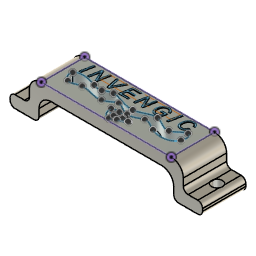
Handle (Autodesk Fusion 360 design; units mm, degrees)
part number: 2025-07-22-14-27-28-106
Autodesk Fusion 360 part; units mm, degrees
note: some values were not read from the file. Chosen so that the rebuilt part matches the saved one: which bodies a step acts on. Set by a fixed rule: which sketch regions a step uses.
sketch "Sketch1" plane through (0, 0, 0) normal (0, 1, 0) x (1, 0, 0)
  line L0 (-40, -2) -> (-40, -3)
  line L1 (-38, -5) -> (-34, -5)
  line L2 (-32, -7) -> (-32, -10)
  line L3 (-27, -15) -> (0.0378, -15)
  line L4 (0, -1.75) -> (0, -22.5)
  line L5 (0, 0) -> (38, 0)
  line L6 (40, -2) -> (40, -3)
  line L7 (38, -5) -> (34, -5)
  line L8 (32, -7) -> (32, -10)
  line L9 (27, -15) -> (-0.0378, -15)
  line L10 (-38, 0) -> (-30, 0)
  line L11 (-28, -2) -> (-28, -5)
  line L12 (-23, -10) -> (0, -10)
  line L13 (40, 0) -> (30, 0)
  line L14 (28, -2) -> (28, -5)
  line L15 (23, -10) -> (0, -10)
  arc A0 (-32, -10) -> (-27, -15) centre (-27, -10) ccw
  arc A1 (27, -15) -> (32, -10) centre (27, -10) ccw
  arc A2 (-28, -5) -> (-23, -10) centre (-23, -5) ccw
  arc A3 (23, -10) -> (28, -5) centre (23, -5) ccw
  arc A4 (-38, 0) -> (-40, -2) centre (-38, -2) ccw
  arc A5 (40, -2) -> (38, 0) centre (38, -2) ccw
  arc A6 (38, -5) -> (40, -3) centre (38, -3) ccw
  arc A7 (30, 0) -> (28, -2) centre (30, -2) ccw
  arc A8 (-28, -2) -> (-30, 0) centre (-30, -2) ccw
  arc A9 (-32, -7) -> (-34, -5) centre (-34, -7) ccw
  arc A10 (34, -5) -> (32, -7) centre (34, -7) ccw
  arc A11 (-40, -3) -> (-38, -5) centre (-38, -3) ccw
  point P0 (-40, 0)
  point P1 (-40, -5)
  point P2 (-32, -5)
  point P3 (-32, -15)
  point P4 (-28, 0)
  dimension "d7" = 40
  dimension "d8" = 5
  dimension "d9" = 8
  dimension "d10" = 10
  dimension "d18" = 12
  dimension "d41" = 5
  dimension "d53" = 5
  dimension "d54" = 5
  dimension "d55" = 2
  dimension "d56" = 2
  constraint perpendicular L0 L1
  constraint perpendicular L1 L2
  constraint perpendicular L2 L3
  constraint symmetric L3.end L4 L9.end
  constraint perpendicular L0 L10
  constraint perpendicular L10 L11
  constraint coincident L4 L12.end
  constraint perpendicular L4 L12
  constraint symmetric P0 L4 L13.start
  constraint symmetric L4 L12.end L15.end
  constraint coincident P3 L2
  constraint coincident P3 L3
  constraint tangent L2 A0
  constraint tangent L3 A0
  constraint symmetric L4 L2.end L8.end
  constraint symmetric L4 L3.start L9.start
  constraint symmetric L4 A0 A1
  constraint tangent L11 A2
  constraint tangent L12 A2
  constraint tangent L14 A3
  constraint tangent L15 A3
  constraint equal A2 A3
  constraint coincident P0 L0
  constraint coincident P0 L10
  constraint tangent L0 A4
  constraint tangent L10 A4
  constraint tangent L5 A5
  constraint tangent L6 A5
  constraint equal A4 A5
  constraint tangent L6 A6
  constraint tangent L7 A6
  constraint equal A4 A6
  constraint tangent L13 A7
  constraint tangent L14 A7
  constraint equal A4 A7
  constraint coincident P4 L10
  constraint coincident P4 L11
  constraint tangent L10 A8
  constraint tangent L11 A8
  constraint equal A4 A8
  constraint coincident P2 L1
  constraint coincident P2 L2
  constraint tangent L1 A9
  constraint tangent L2 A9
  constraint equal A4 A9
  constraint tangent L7 A10
  constraint tangent L8 A10
  constraint equal A4 A10
  constraint coincident P1 L0
  constraint coincident P1 L1
  constraint tangent L0 A11
  constraint tangent L1 A11
  measures "d7" distance of L5.start P0
  measures "d8" distance of P0 P1
  measures "d9" distance of P1 P2
  measures "d10" distance of P2 P3
  measures "d18" distance of P0 P4
  measures "d41" distance of L3 L12
  measures "d53" radius of A0
  measures "d54" radius of A2
  measures "d55" radius of A4
  measures "d56" radius of A11
extrude "Extrude2" add sketch "Sketch1" along normal blind 18 makes body 1
sketch "Sketch3" plane through (0, 0, 15) normal (0, 0, 1) x (-1, 0, 0)
  line L0 (27, 0) -> (-27, 0)
  line L1 (-27, -18) -> (27, -18)
  line L2 (15.4669, -13.2004) -> (-13.5401, -13.4911) construction
  line L3 (-13.5401, -13.4911) -> (-13.5035, -17.1453) construction
  line L4 (-13.5035, -17.1453) -> (15.5035, -16.8547) construction
  line L5 (15.5035, -16.8547) -> (15.4669, -13.2004) construction
  spline S0 degree 5 poles (3, -5) (3, -4.7009) (2.9694, -4.1277) (2.8315, -3.3428) (2.4733, -2.45) (1.7882, -1.6139) (0.9367, -1.0903) (0, -0.9102) (-0.9367, -1.0903) (-1.7882, -1.6139) (-2.4733, -2.45) (-2.8315, -3.3428) (-2.9694, -4.1277) (-3, -4.7009) (-3, -5) knots 0 0 0 0 0 0 0.1 0.2 0.3 0.4 0.5 0.6 0.7 0.8 0.9 1 1 1 1 1 1
  line L6 (3, -6) -> (3, -4)
  line L7 (-3, -4) -> (-3, -6)
  spline S1 degree 5 poles (3, -5) (3.0104, -4.9295) (3.0012, -4.7732) (2.8966, -4.496) (2.5814, -4.0664) (1.9381, -3.5344) (1.1107, -3.1246) (0.179, -2.9363) (-0.7694, -3.0239) (-1.6457, -3.3607) (-2.3664, -3.8604) (-2.8601, -4.409) (-3.0745, -4.894) (-2.983, -5.2313) (-2.5948, -5.4017) (-1.9522, -5.4436) (-1.1205, -5.4206) (-0.1814, -5.3963) (0.7751, -5.4088) (1.6575, -5.4391) (2.3801, -5.4296) (2.7723, -5.3367) (2.9386, -5.1964) (2.9896, -5.0705) (3, -5) knots 0 0 0 0 0 0 0.05 0.1 0.15 0.2 0.25 0.3 0.35 0.4 0.45 0.5 0.55 0.6 0.65 0.7 0.75 0.8 0.85 0.9 0.95 1 1 1 1 1 1
  spline S2 degree 5 poles (-1.9403, -1.8799) (-2.1918, -1.9781) (-2.6753, -2.1699) (-3.3422, -2.4439) (-4.1125, -2.7815) (-4.8632, -3.1539) (-5.3805, -3.4718) (-5.6414, -3.7297) (-5.6271, -3.9233) (-5.3382, -4.0528) (-4.7908, -4.1218) (-4.161, -4.1322) (-3.5872, -4.1163) (-3.1604, -4.0953) (-2.9358, -4.0822) knots 0 0 0 0 0 0 0.1 0.2 0.3 0.4 0.5 0.6 0.7 0.8 0.9 1 1 1 1 1 1
  spline S3 degree 5 poles (-2.8985, -3.8613) (-3.0894, -3.8838) (-3.4527, -3.9238) (-3.9421, -3.9686) (-4.4817, -3.9973) (-4.9558, -3.9783) (-5.2137, -3.8999) (-5.2411, -3.7584) (-5.0366, -3.5532) (-4.6152, -3.2885) (-3.996, -2.9697) (-3.3566, -2.675) (-2.8014, -2.4333) (-2.3982, -2.2631) (-2.1883, -2.1758) knots 0 0 0 0 0 0 0.1 0.2 0.3 0.4 0.5 0.6 0.7 0.8 0.9 1 1 1 1 1 1
  spline S4 degree 5 poles (24, -10) (24.1007, -9.8128) (24.2421, -9.4089) (24.2736, -8.7291) (23.9832, -7.7567) (23.2223, -6.6823) (22.246, -5.9721) (21.2086, -5.7534) (20.1688, -5.9682) (19.1065, -6.422) (17.9657, -6.874) (16.6858, -7.1078) (15.2422, -7.0221) (13.6694, -6.6775) (12.0353, -6.2257) (10.4251, -5.8606) (8.9202, -5.7585) (7.5816, -6.0278) (6.4268, -6.6425) (5.4217, -7.4223) (4.503, -8.1248) (3.5967, -8.5199) (2.636, -8.4636) (1.5834, -7.9922) (0.4311, -7.2894) (-0.8067, -6.5998) (-2.0991, -6.1579) (-3.4049, -6.1167) (-4.6777, -6.4602) (-5.8758, -7.0406) (-6.9721, -7.648) (-7.9648, -8.0702) (-8.8869, -8.1555) (-9.818, -7.877) (-10.8576, -7.3049) (-12.0966, -6.5717) (-13.5903, -5.8414) (-15.3282, -5.2756) (-17.2136, -5.0044) (-19.0984, -5.119) (-20.8113, -5.6611) (-22.1877, -6.6145) (-23.1001, -7.8947) (-23.4868, -9.3402) (-23.3838, -10.7005) (-22.8905, -11.7071) (-22.1322, -12.1498) (-21.2247, -11.9466) (-20.2344, -11.2288) (-19.1882, -10.2675) (-18.0886, -9.3812) (-16.9271, -8.8522) (-15.6985, -8.8353) (-14.4138, -9.2798) (-13.0928, -10.004) (-11.758, -10.7601) (-10.4279, -11.3051) (-9.1114, -11.4623) (-7.7994, -11.204) (-6.4688, -10.6351) (-5.0913, -9.933) (-3.6404, -9.3021) (-2.1001, -8.9215) (-0.4719, -8.8968) (1.2169, -9.2071) (2.9203, -9.7414) (4.5826, -10.3394) (6.1459, -10.8299) (7.5585, -11.072) (8.7831, -10.9905) (9.8052, -10.6266) (10.6384, -10.1184) (11.3305, -9.6367) (11.9652, -9.338) (12.6728, -9.3012) (13.5974, -9.5264) (14.8466, -9.9542) (16.448, -10.4791) (18.3004, -10.9643) (20.2165, -11.2665) (21.9696, -11.2613) (23.065, -10.9472) (23.6377, -10.5323) (23.8993, -10.1872) (24, -10) knots 0 0 0 0 0 0 0.0125 0.025 0.0375 0.05 0.0625 0.075 0.0875 0.1 0.1125 0.125 0.1375 0.15 0.1625 0.175 0.1875 0.2 0.2125 0.225 0.2375 0.25 0.2625 0.275 0.2875 0.3 0.3125 0.325 0.3375 0.35 0.3625 0.375 0.3875 0.4 0.4125 0.425 0.4375 0.45 0.4625 0.475 0.4875 0.5 0.5125 0.525 0.5375 0.55 0.5625 0.575 0.5875 0.6 0.6125 0.625 0.6375 0.65 0.6625 0.675 0.6875 0.7 0.7125 0.725 0.7375 0.75 0.7625 0.775 0.7875 0.8 0.8125 0.825 0.8375 0.85 0.8625 0.875 0.8875 0.9 0.9125 0.925 0.9375 0.95 0.9625 0.975 0.9875 1 1 1 1 1 1
  line L8 (-27, 0) -> (-27, -18)
  line L9 (27, -18) -> (27, 0)
  point P0 (0, -1)
  point P1 (0, -3)
  point P2 (-0.0022, -5.4045)
  point P3 (-5.6, -3.8)
  point P4 (-5.2, -3.8)
  point P5 (22, -6)
  point P6 (17, -7)
  point P7 (8, -6)
  point P8 (3.3028, -8.4387)
  point P9 (-2.386, -6.2141)
  point P10 (-8, -8)
  point P11 (-13.3822, -5.9916)
  point P12 (-23, -8)
  point P13 (-22, -12)
  point P14 (-17, -9)
  point P15 (-10.0134, -11.299)
  point P16 (-2, -9)
  point P17 (8, -11)
  point P18 (11.5023, -9.5829)
  point P19 (15, -10)
  dimension "d45" = 5
  text T0 "INVENGIC" font "Arial" height 5 italic align centre top in box 29.0085 x 3.6544 at (15.4669, -13.2004) x (-0.99995, -0.01002) y (0.01002, -0.99995) spacing 1.5
  constraint midpoint S0.start L6
  constraint midpoint S0.end L7
  constraint coincident S0 S2.start
  constraint coincident S0 S2.end
  constraint coincident S0 S3.start
  constraint coincident S0 S3.end
sketch "Sketch4" plane through (0, 0, 5) normal (0, 0, 1) x (-1, 0, 0)
  circle A0 centre (36, -10) radius 2.25
  line L0 (0, -1.75) -> (0, -22.5)
  circle A1 centre (-36, -10) radius 2.25
  line L1 (38, 0) -> (34, 0)
  line L2 (34, -18) -> (38, -18)
  line L3 (34, 0) -> (34, -18)
  line L4 (38, -18) -> (38, 0)
  dimension "d28" = 4.5
  constraint symmetric A0 L0 A1
  measures "d28" diameter of A0
extrude "Extrude4" cut sketch "Sketch4" against normal blind 9 contours A0 L4 | A0 L3 L4 | A0 L3 | A1 bodies 1
extrude "Extrude6" cut sketch "Sketch3" against normal through all text T0 bodies 1
extrude "Extrude7" cut sketch "Sketch3" against normal blind 7 contours S0 S1 | S0 S2 S3 | S0 L6 L7 S1 bodies 1 makes body 2 at (-15.1678, 5.0678, 15)
extrude "Extrude8" cut sketch "Sketch3" against normal through all contours S4 bodies 2
